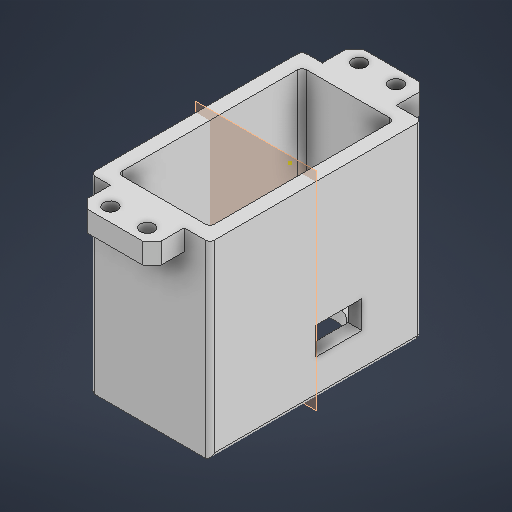
# Autodesk Inventor part: servo_holder
Saved by Autodesk Inventor 2026 (Build 300175050, 175E)
## iProperties
Created: 2025-05-22
Part Number: servo_holder
Material: Generic
Document SubType Name: Modeling
Designer: sumit
Density: 1 g/cm^3
Appearance: Default
Author: sumit
Autodesk Inventor part; units mm, degrees
ref_plane "YZ Plane" through (0, 0, 0) normal (1, 0, 0) x (0, 1, 0)
ref_plane "XZ Plane" through (0, 0, 0) normal (0, 1, 0) x (-1, 0, 0)
ref_plane "XY Plane" through (0, 0, 0) normal (0, 0, 1) x (1, 0, 0)
sketch "Sketch1" plane through (0, 0, 0) normal (0, 1, 0) x (-1, 0, 0)
  line L0 (12.0626, 25.212) -> (-7.9374, 25.212)
  line L1 (-7.9374, 25.212) -> (-7.9374, -14.788)
  line L2 (-7.9374, -14.788) -> (12.0626, -14.788)
  line L3 (12.0626, -14.788) -> (12.0626, 25.212)
  line L4 (12.0626, 25.212) -> (-7.9374, -14.788) construction
  line L5 (-7.9374, 25.212) -> (12.0626, -14.788) construction
  point P0 (0, 0)
  point P1 (2.0626, 5.212)
  dimension "d0" = 20
  dimension "d1" = 40
  constraints: 12 end point, 2 midpoint, 2 parallel, 1 horizontal, 1 perpendicular
  measures "d0" distance of L2.end L1.end
  measures "d1" distance of L1.end L0.end
extrude "Extrusion1" add sketch "Sketch1" along normal blind 3
sketch "Sketch2" plane through (0, 3, 0) normal (0, 1, 0) x (1, 0, 0)
  line L0 (-15.0626, -28.212) -> (10.9374, -28.212)
  line L1 (10.9374, -28.212) -> (10.9374, 17.788)
  line L2 (10.9374, 17.788) -> (-15.0626, 17.788)
  line L3 (-15.0626, 17.788) -> (-15.0626, -28.212)
  line L4 (-15.0626, -28.212) -> (10.9374, 17.788) construction
  line L5 (10.9374, -28.212) -> (-15.0626, 17.788) construction
  line L6 (-12.0626, 14.788) -> (-12.0626, -25.212) projected
  line L7 (-12.0626, -25.212) -> (7.9374, -25.212) projected
  line L8 (7.9374, 14.788) -> (-12.0626, 14.788)
  line L9 (-12.0626, 14.788) -> (-12.0626, -25.212)
  line L10 (-12.0626, -25.212) -> (7.9374, -25.212)
  line L11 (7.9374, -25.212) -> (7.9374, 14.788)
  line L12 (7.9374, 14.788) -> (-12.0626, -25.212) construction
  line L13 (-12.0626, 14.788) -> (7.9374, -25.212) construction
  point P0 (0, 0)
  point P1 (-2.0626, -5.212)
  point P2 (7.9374, -25.212)
  dimension "d4" = 26
  dimension "d5" = 46
  dimension "d6" = 3
  dimension "d7" = 3
  constraints: 24 end point, 4 midpoint, 4 parallel, 2 horizontal, 2 perpendicular
  measures "d4" distance of L2.end L1.end
  measures "d5" distance of L1.end L0.end
  measures "d6" distance between parallel lines of L6 L3
  measures "d7" distance between parallel lines of L0 L7
extrude "Extrusion2" add sketch "Sketch2" along normal blind 38 and the other way blind 3
fillet "Fillet1" radius 1 13 edges at (10.9374, 0, 5.212) (-2.0626, 0, -17.788) (10.9374, 20.5, -17.788) (-15.0626, 20.5, -17.788) (-15.0626, 0, 5.212) (10.9374, 20.5, 28.212) (-15.0626, 20.5, 28.212) (-12.0626, 22, -14.788) (-12.0626, 3, 5.212) (7.9374, 3, 5.212) (7.9374, 22, -14.788) (7.9374, 22, 25.212) (-12.0626, 22, 25.212)
sketch "Sketch8" plane through (10.9374, 1, 27.212) normal (1, 0, 0) x (0, 0, -1)
  line L0 (32, 7) -> (22, 7)
  line L1 (22, 7) -> (22, 13)
  line L2 (22, 13) -> (32, 13)
  line L3 (32, 13) -> (32, 7)
  line L4 (-1, -1) -> (44, -1) projected
  line L5 (45, 0) -> (45, 40) projected
  point P0 (27.212, -1)
  point P1 (27, 7)
  dimension "d25" = 10
  dimension "d26" = 6
  dimension "d27" = 8
  dimension "d28" = 13
  constraints: 8 end point, 2 parallel, 1 horizontal, 1 midpoint, 1 perpendicular
  measures "d25" distance of L1.end L2.end
  measures "d26" distance of L0.end L1.end
  measures "d27" distance from line of point (27, 7) L4
  measures "d28" distance between parallel lines of L5 L3
extrude "Extrusion4" cut sketch "Sketch8" against normal blind 3
sketch "Sketch9" plane through (0, 0, 0) normal (0, -1, 0) x (1, 0, 0)
  circle A0 centre (-2.0626, -5.288) radius 6.5
  line L0 (-14.0626, -17.788) -> (9.9374, -17.788) projected
  line L1 (10.9374, -16.788) -> (10.9374, 27.212) projected
  point P0 (0, 0)
  dimension "d31" = 13
  dimension "d32" = 12.5
  dimension "d36" = 13
  constraints: 1 centre point
  measures "d31" diameter of A0
  measures "d32" distance from line of L0 A0.centre
  measures "d36" distance from line of L1 A0.centre
extrude "Extrusion5" cut sketch "Sketch9" against normal blind 3
sketch "Sketch11" plane through (-14.0626, 0, 28.212) normal (0, 0, 1) x (1, 0, 0)
  line L0 (19.4055, 36.5) -> (3.4055, 36.5)
  line L1 (3.4055, 36.5) -> (3.4055, 41)
  line L2 (3.4055, 41) -> (19.4055, 41)
  line L3 (19.4055, 41) -> (19.4055, 36.5)
  line L4 (0, 41) -> (24, 41) projected
  point P0 (14.0626, 0)
  point P1 (11.4055, 41)
  dimension "d37" = 16
  dimension "d38" = 4.5
  dimension "d39" = 0
  constraints: 8 end point, 2 parallel, 1 horizontal, 1 midpoint, 1 perpendicular
  measures "d37" distance of L0.start L0.end
  measures "d38" distance of L2.end L0.start
  measures "d39" distance from line of point (11.405, 41) L4
extrude "Extrusion6" add sketch "Sketch11" along normal blind 7
chamfer "Chamfer1" distance 2 angle 45 2 edges at (-10.6572, 38.75, 35.212) (5.3428, 38.75, 35.212)
sketch "Sketch12" plane through (-10.6572, 36.5, 28.212) normal (0, -1, 0) x (1, 0, 0)
  point P0 (10.6572, -28.212)
sketch "Sketch13" plane through (-10.6572, 36.5, 28.212) normal (0, -1, 0) x (1, 0, 0)
  circle A0 centre (12, 4) radius 1.5
  circle A1 centre (4, 4) radius 1.5
  line L0 (16, 0) -> (16, 5) projected
  line L1 (2, 7) -> (14, 7) projected
  line L2 (0, 0) -> (0, 5) projected
  point P0 (10.6572, -28.212)
  dimension "d45" = 3
  dimension "d46" = 3
  dimension "d47" = 4
  dimension "d48" = 3
  dimension "d49" = 4
  dimension "d50" = 3
  constraints: 2 centre point
  measures "d45" diameter of A0
  measures "d46" diameter of A1
  measures "d47" distance from line of L0 A0.centre
  measures "d48" distance from line of L1 A0.centre
  measures "d49" distance from line of L2 A1.centre
  measures "d50" distance from line of L1 A1.centre
extrude "Extrusion7" cut sketch "Sketch13" against normal blind 7
ref_plane "Work Plane1" through (-14.0626, 0, 5.212) normal (0, 0, 1) x (1, 0, 0)
mirror "Mirror1" about plane through (-14.0626, 0, 5.212) normal (0, 0, 1) of "Extrusion6", "Extrusion7", "Chamfer1"
body "Solid1"
